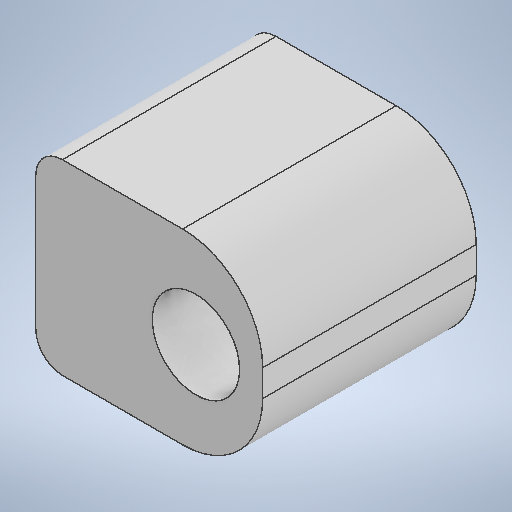
# Autodesk Inventor part: spacer_link
Saved by Autodesk Inventor 2025 (Build 290162000, 162)
## iProperties
Created: 2025-12-09
Part Number: spacer_link
Material: 一般
Document SubType Name: Modeling
Designer: sooo1
Density: 1 g/cm^3
Appearance: 既定
Author: sooo1
Autodesk Inventor part; units mm, degrees
ref_plane "YZ Plane" through (0, 0, 0) normal (1, 0, 0) x (0, 1, 0)
ref_plane "XZ Plane" through (0, 0, 0) normal (0, 1, 0) x (-1, 0, 0)
ref_plane "XY Plane" through (0, 0, 0) normal (0, 0, 1) x (1, 0, 0)
sketch "スケッチ1" plane through (0, 0, 0) normal (0, 0, 1) x (1, 0, 0)
  line L0 (-4.25, 3.5) -> (1.25, 3.5)
  line L1 (4.25, 0.5) -> (4.25, -0.5)
  line L2 (1.25, -3.5) -> (-4.25, -3.5)
  line L3 (-4.25, -3.5) -> (-4.25, 3.5)
  line L4 (-4.25, 3.5) -> (4.25, -3.5) construction
  line L5 (4.25, 3.5) -> (-4.25, -3.5) construction
  arc A0 (4.25, 0.5) -> (1.25, 3.5) centre (1.25, 0.5) ccw
  arc A1 (1.25, -3.5) -> (4.25, -0.5) centre (1.25, -0.5) ccw
  circle A2 centre (1.75, 0) radius 1.635
  line L6 (-6.0743, 0) -> (6.6956, 0) construction
  point P0 (0, 0)
  dimension "d0" = 7
  dimension "d1" = 8.5
  dimension "d2" = 3
  dimension "d6" = 3.27
  dimension "d7" = 2.5
  constraints: 12 end point, 5 point on line, 4 point on circle, 4 tangent, 3 centre point, 2 midpoint, 2 parallel, 1 equal radius, 1 horizontal, 1 perpendicular
  measures "d0" distance of L2.end L0.start
  measures "d1" distance of L0.start L5.start
  measures "d2" radius of A0
  measures "d6" diameter of A2
  measures "d7" distance from line of L1 A2.centre
extrude "押し出し1" add sketch "スケッチ1" along normal blind 8
fillet "フィレット1" radius 1 2 edges at (-4.25, 3.5, 4) (-4.25, -3.5, 4)
